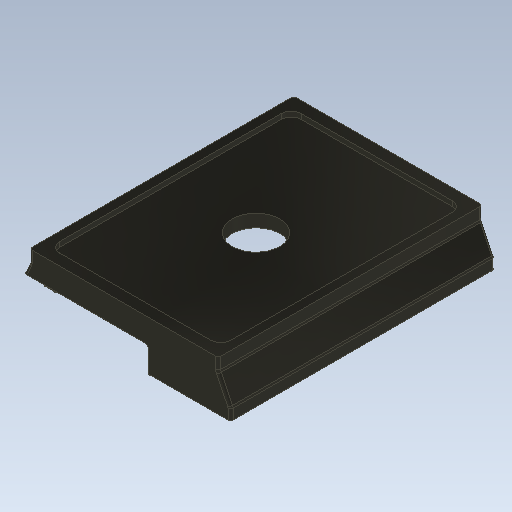
# Autodesk Inventor part: Quick Release Mounting
Saved by Autodesk Inventor 2020 (Build 240168000, 168)
## iProperties
Created: 2012-10-13
Part Number: Quick Release Mounting
Document SubType Name: Modeling
Designer: Lance
Density: 7.85 g/cm^3
Material: Steel, Mild
Mass: 82.2062 g
Surface Area: 62.6778 cm^2
Volume: 10.4721 cm^3
Appearance: Gunmetal
Author: Lance
Autodesk Inventor part; units mm, degrees
ref_plane "YZ Plane" through (0, 0, 0) normal (1, 0, 0) x (0, 1, 0)
ref_plane "XZ Plane" through (0, 0, 0) normal (0, 1, 0) x (-1, 0, 0)
ref_plane "XY Plane" through (0, 0, 0) normal (0, 0, 1) x (1, 0, 0)
sketch "Sketch1" plane through (0, 0, 0) normal (0, 0, 1) x (1, 0, 0)
  line L0 (-21.2, -5) -> (-21.2, -2.5)
  line L1 (-21.2, -2.5) -> (-18.75, 2.5)
  line L2 (-18.75, 2.5) -> (-18.75, 5)
  line L3 (-18.75, 5) -> (18.75, 5)
  line L4 (18.75, 5) -> (18.75, 2.5)
  line L5 (18.75, 2.5) -> (21.2, -2.5)
  line L6 (21.2, -2.5) -> (21.2, -5)
  line L7 (21.2, -5) -> (-21.2, -5)
  line L8 (0, -7) -> (0, 7) projected
  point P0 (0, 0)
  dimension "d0" = 2.5
  dimension "d1" = 2.5
  dimension "d2" = 10
  dimension "d3" = 37.5
  dimension "d4" = 42.4
  dimension "d5" = 5
  constraints: 16 end point, 3 parallel, 2 perpendicular, 1 vertical, 3 other
  measures "d0" distance from line of L3 L1.end
  measures "d1" distance of L0.start L0.end
  measures "d2" distance between parallel lines of L7 L3
  measures "d3" distance between parallel lines of L4 L2
  measures "d4" distance between parallel lines of L6 L0
  measures "d5" distance from line of point (0, 0) L3
extrude "Extrusion1" add sketch "Sketch1" along normal mid plane 52.5
sketch "Sketch2" plane through (-21.2, -5, 26.25) normal (0, -1, 0) x (1, 0, 0)
  line L0 (3, -3) -> (39.4, -3)
  line L1 (39.4, -3) -> (39.4, -49.5)
  line L2 (39.4, -49.5) -> (3, -49.5)
  line L3 (3, -49.5) -> (3, -3)
  line L4 (42.4, 0) -> (0, 0) projected
  line L5 (42.4, 0) -> (42.4, -52.5) projected
  point P0 (21.2, -26.25)
  point P1 (21.2, -3)
  point P2 (3, -26.25)
  dimension "d8" = 3
  dimension "d9" = 3
  constraints: 8 end point, 2 midpoint, 2 parallel, 1 horizontal, 1 horizontal alignment, 1 perpendicular, 1 vertical alignment
  measures "d8" distance between parallel lines of L4 L0
  measures "d9" distance between parallel lines of L5 L1
extrude "Extrusion2" cut sketch "Sketch2" against normal up to surface (5 mm away) draft -30
sketch "Sketch3" plane through (0, 0, 26.25) normal (0, 0, 1) x (1, 0, 0)
  line L0 (-21.2, -2.5) -> (-18.75, 2.5) projected
  line L1 (-21.2, -5) -> (-21.2, -2.5) projected
  line L2 (21.2, -5) -> (-21.2, -5) projected
  line L3 (21.2, -2.5) -> (21.2, -5) projected
  line L4 (18.75, 2.5) -> (21.2, -2.5) projected
  line L5 (18.75, 5) -> (18.75, 2.5) projected
  line L6 (-18.75, 5) -> (18.75, 5) projected
  line L7 (-18.75, 2.5) -> (-18.75, 5) projected
  line L8 (15.3132, 0) -> (-15.3132, 0) projected
  line L9 (-19.975, 0) -> (4.7, 0)
  line L10 (4.7, 0) -> (4.7, -5)
  point P0 (0, 0)
  dimension "d12" = 16.5
  constraints: 4 end point, 2 collinear, 1 midpoint, 1 perpendicular, 1 point on line
  measures "d12" distance between parallel lines of L3 L10
extrude "Extrusion3" cut sketch "Sketch3" against normal blind 4.85 contours L0 L9 L8 L10 L2 L1
mirror "Mirror1" about plane through (0, 0, 0) normal (0, 0, 1) of "Extrusion3"
sketch "Sketch4" plane through (4.7, 0, -21.4) normal (0, 0, -1) x (-1, 0, 0)
  line L0 (22.9, -5) -> (20.0132, 0)
  line L1 (20.0132, 0) -> (0, 0)
  line L2 (0, 0) -> (0, -5)
  line L3 (0, -5) -> (22.9, -5)
  line L4 (-13.5, -5) -> (0, -5) projected
  line L5 (0, 0) -> (24.675, 0) projected
  line L6 (0, -1.7957) -> (0, 0) projected
  line L7 (22.9, -5) -> (21.05, -1.7957) projected
  point P0 (4.7, 0)
  constraints: 8 end point, 4 collinear, 2 perpendicular, 1 horizontal
extrude "Extrusion4" cut sketch "Sketch4" against normal through all
fillet "Fillet1" radius 3 2 edges at (16.7566, -2.5, 21.8066) (16.7566, -2.5, -21.8066)
fillet "Fillet2" radius 1 4 edges at (-18.75, 2.5, 0) (-21.2, -2.5, 0) (18.75, 2.5, 0) (21.2, -2.5, 0)
fillet "Fillet3" radius 0.5 22 edges at (-18.75, 3.8659, 26.25) (-18.7758, 2.506, 26.25) (-19.4135, 1.1459, 26.25) (18.75, 3.8659, 26.25) (18.7758, 2.506, 26.25) (19.975, 0, 26.25) (21.1742, -2.506, 26.25) (21.2, -3.8659, 26.25) (18.75, 3.8659, -26.25) (18.7758, 2.506, -26.25) (19.975, 0, -26.25) (21.1742, -2.506, -26.25) (21.2, -3.8659, -26.25) (-18.75, 3.8659, -26.25) (-18.7758, 2.506, -26.25) (-19.4135, 1.1459, -26.25) (-20.5365, -1.1459, 21.4) (-21.1742, -2.506, 21.4) (-21.2, -3.8659, 21.4) (-20.5365, -1.1459, -21.4) (-21.1742, -2.506, -21.4) (-21.2, -3.8659, -21.4)
fillet "Fillet5" radius 3 6 edges at (-15.3132, 0, 0) (15.3132, 0, 0) (14.5878, 0, 19.6378) (8.7076, 0, 20.3632) (14.5878, 0, -19.6378) (8.7076, 0, -20.3632)
fillet "Fillet4" radius 0.5 4 edges at (-17.1896, -3.25, 21.4) (-17.1896, -3.25, -21.4) (4.7, -3.25, -22.2396) (4.7, -3.25, 22.2396)
fillet "Fillet6" radius 0.5 10 edges at (-17.4011, 0, 21.4) (-19.8119, 0, 21.2536) (-14.4858, 0, 21.24) (4.7, 0, 23.342) (4.86, 0, 19.5358) (4.7, 0, -23.342) (4.86, 0, -19.5358) (-14.4858, 0, -21.24) (-17.4011, 0, -21.4) (-19.8119, 0, -21.2536)
fillet "Fillet7" radius 0.25 8 edges at (-21.2, -5, 0) (-21.0536, -5, 21.2536) (-19.7387, -5, 21.4) (-18.3691, -5, 21.2536) (-18.2, -5, 0) (-18.3691, -5, -21.2536) (-19.7387, -5, -21.4) (-21.0536, -5, -21.2536)
fillet "Fillet8" radius 0.25 12 edges at (4.7, -2.75, 26.25) (4.5536, -0.1464, 26.25) (-7.6091, 0, 26.25) (-19.8119, 0, 26.1036) (-19.975, 0, 23.7935) (-20.1061, -0.2676, 21.3147) (4.7, -2.75, -26.25) (4.5536, -0.1464, -26.25) (-7.6091, 0, -26.25) (-19.8119, 0, -26.1036) (-19.975, 0, -23.7935) (-20.1061, -0.2676, -21.3147)
fillet "Fillet9" radius 0.25 16 edges at (4.7, -5, 24.9137) (4.8464, -5, 23.4191) (10.401, -5, 23.25) (17.4745, -5, 22.5245) (18.2, -5, 0) (17.4745, -5, -22.5245) (10.401, -5, -23.25) (4.8464, -5, -23.4191) (4.7, -5, -24.9137) (4.7732, -5, -26.1768) (12.825, -5, -26.25) (21.0536, -5, -26.1036) (21.2, -5, 0) (21.0536, -5, 26.1036) (12.825, -5, 26.25) (4.7732, -5, 26.1768)
sketch "Sketch5" plane through (-18.25, 5, 26.25) normal (0, 1, 0) x (1, 0, 0)
  line L0 (1.25, 50.25) -> (35.25, 50.25)
  line L1 (35.25, 50.25) -> (35.25, 2.25)
  line L2 (35.25, 2.25) -> (1.25, 2.25)
  line L3 (1.25, 2.25) -> (1.25, 50.25)
  point P0 (18.25, 26.25)
  point P1 (1.25, 26.25)
  point P2 (18.25, 50.25)
  dimension "d26" = 34
  dimension "d27" = 48
  constraints: 8 end point, 2 midpoint, 2 parallel, 1 horizontal, 1 horizontal alignment, 1 perpendicular, 1 vertical alignment
  measures "d26" distance between parallel lines of L1 L3
  measures "d27" distance between parallel lines of L2 L0
extrude "Extrusion5" cut sketch "Sketch5" against normal blind 1
fillet "Fillet10" radius 2 4 edges at (-17, 4.5, -24) (17, 4.5, -24) (-17, 4.5, 24) (17, 4.5, 24)
sketch "Sketch6" plane through (13.5812, 0, -18.6312) normal (0, -1, 0) x (1, 0, 0)
  circle A0 centre (-13.5812, 18.6312) radius 7.75
  dimension "d31" = 15.5
  constraints: 1 centre point, 1 coincident
  measures "d31" diameter of A0
extrude "Extrusion6" cut sketch "Sketch6" against normal blind 1.5
sketch "Sketch7" plane through (0, 1.5, 0) normal (0, -1, 0) x (1, 0, 0)
  circle A0 centre (0, 0) radius 4.75
  dimension "d34" = 9.5
  constraints: 1 centre point, 1 coincident
  measures "d34" diameter of A0
extrude "Extrusion7" cut sketch "Sketch7" against normal through all
body "Solid1"
